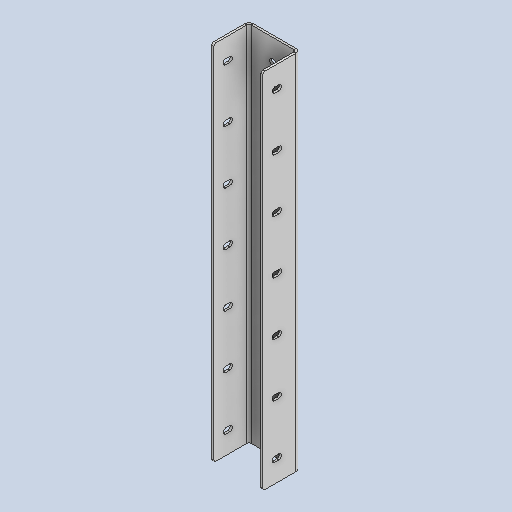
# Autodesk Inventor part: NDM 4.0.5  mother bottom
Saved by Autodesk Inventor 2025 (Build 290162010, 162A)
## iProperties
Created: 2023-07-04
Part Number: NDM 4.0.5  mother bottom
Material: Stainless Steel
Document SubType Name: Sheet Metal
Designer: user
Density: 8 g/cm^3
Sheet Metal Rule: Default_mm
Appearance: Default
Flat Pattern Width: 11.1048 cm
Flat Pattern Length: 34 cm
Flat Pattern Area: 377.562 cm^2
Sheet Metal Width: 111.048 mm
Sheet Metal Length: 340.000 mm
Sheet Metal Area: 37756.248 mm^2
Description: 2mm
Stock Number: NDM 4.0.5 мама низ
Mass: 594.459 g
Surface Area: 770.179 cm^2
Volume: 74.3073 cm^3
Author: user
Revision Number: 8
Autodesk Inventor part; units mm, degrees
ref_plane "YZ Plane" through (0, 0, 0) normal (1, 0, 0) x (0, 1, 0)
ref_plane "XZ Plane" through (0, 0, 0) normal (0, 1, 0) x (-1, 0, 0)
ref_plane "XY Plane" through (0, 0, 0) normal (0, 0, 1) x (1, 0, 0)
sketch "Sketch1" plane through (0, 0, 0) normal (0, 0, 1) x (1, 0, 0)
  line L0 (-22, 340) -> (22, 340)
  line L1 (22, 340) -> (22, 0)
  line L2 (22, 0) -> (-22, 0)
  line L3 (-22, 0) -> (-22, 340)
  line L4 (-22, 340) -> (22, 0) construction
  line L5 (22, 340) -> (-22, 0) construction
  point P0 (0, 0)
  point P1 (0, 170)
  point P2 (0, 0)
  dimension "d0" = 44
  dimension "d1" = 340
  constraints: 12 end point, 3 midpoint, 2 parallel, 1 coincident, 1 horizontal, 1 perpendicular
  measures "d0" distance of L1.end L2.end
  measures "d1" distance of L2.end L0.start
extrude "Plate1" add sketch "Sketch1" along normal blind 2
sketch "Sketch2" plane through (-22, 0, 2) normal (-1, 0, 0) x (0, -1, 0)
  line L0 (-340, 0) -> (0, 0)
  line L1 (0, 0) -> (0, 33)
  line L2 (0, 33) -> (-340, 33)
  line L3 (-340, 33) -> (-340, 0)
  constraints: 6 end point, 1 horizontal, 1 perpendicular, 1 vertical
edge flange "Flange1" height 35 angle 90 thickness 2 bend radius 2 thickness toward (-1, 0, 0) relief tear relief width 2 relief depth 1 corner gap 2 corner form 0 edges at (-22, 170, 2) (22, 170, 2) wall of the first edge with corners at (-22, 340, 2) (-22, 0, 2) (-22, 0, 35) (-22, 340, 35)
bend "Bend1"
corner "Corner1"
sketch "Sketch3" plane through (0, 0, 0) normal (1, 0, 0) x (0, 1, 0)
  line L0 (0, 4) -> (340, 4) projected
  line L1 (340, 35) -> (340, 4) projected
  line L2 (0, 35) -> (340, 35) projected
  line L3 (0, 4) -> (0, 35) projected
  circle A0 centre (20, 22) radius 2.5
  line L4 (20, 20) -> (20, 24) construction
  line L5 (22.5, 20) -> (22.5, 24)
  line L6 (17.5, 24) -> (17.5, 20)
  arc A1 (17.5, 20) -> (22.5, 20) centre (20, 20) ccw
  arc A2 (22.5, 24) -> (17.5, 24) centre (20, 24) ccw
  point P0 (0, 0)
  point P1 (17.5, 22)
  point P2 (22.5, 22)
  dimension "d13" = 5
  dimension "d14" = 13
  dimension "d15" = 20
  dimension "d28" = 4
  dimension "d29" = 2.5
  constraints: 8 end point, 4 point on circle, 4 tangent, 3 centre point, 1 coincident, 1 midpoint, 1 parallel, 1 vertical
  measures "d13" diameter of A0
  measures "d14" distance from line of A0.centre L2
  measures "d15" distance from line of L3 A0.centre
  measures "d28" distance of L4.start L4.end
  measures "d29" radius of A2
extrude "Extrusion1" cut sketch "Sketch3" along normal through all both and the other way through all contours A0 | L5 A1 L6 A0 | A0 L6 A2 L5
sketch "Sketch4" plane through (0, 0, 0) normal (0, 0, -1) x (-1, 0, 0)
  circle A0 centre (0, 20) radius 2.5
  line L0 (-20, 0) -> (20, 0) projected
  line L1 (-0.5, 20) -> (0.5, 20) construction
  line L2 (-0.5, 17.5) -> (0.5, 17.5)
  line L3 (0.5, 22.5) -> (-0.5, 22.5)
  arc A1 (-0.5, 22.5) -> (-0.5, 17.5) centre (-0.5, 20) ccw
  arc A2 (0.5, 17.5) -> (0.5, 22.5) centre (0.5, 20) ccw
  point P0 (0, 0)
  point P1 (0, 0)
  point P2 (0, 22.5)
  point P3 (0, 17.5)
  dimension "d21" = 5
  dimension "d22" = 20
  dimension "d30" = 1
  dimension "d31" = 5
  constraints: 8 end point, 4 point on circle, 4 tangent, 3 centre point, 2 midpoint, 1 coincident, 1 horizontal, 1 parallel, 1 vertical alignment
  measures "d21" diameter of A0
  measures "d22" distance from line of A0.centre L0
  measures "d30" distance of L1.start L1.end
  measures "d31" diameter of A2
extrude "Extrusion2" cut sketch "Sketch4" against normal through all
pattern_linear "Rectangular Pattern2" count 7 spacing 50 along (0, 1, 0) of "Extrusion2", "Extrusion1"
fillet "Fillet1" radius 2 4 edges at (-23, 0, 35) (23, 0, 35) (-23, 340, 35) (23, 340, 35)
equation "\"d22\" = d15"
equation "\"d2\" = Thickness"
equation "\"d3\" = BendReliefWidth"
equation "\"d4\" = BendReliefDepth"
equation "\"d5\" = MinimumRemnant"
equation "\"d6\" = TransitionRadius"
equation "\"d9\" = BendRadius"
equation "\"d10\" = CornerReliefSize"
equation "\"d11\" = GapSize"
equation "\"d12\" = JacobiRadiusSize"
equation "\"BendRadius\" = Thickness"
equation "\"BendReliefWidth\" = Thickness"
equation "\"BendReliefDepth\" = 0.5 * Thickness"
equation "\"CornerReliefSize\" = 4 * Thickness"
equation "\"MinimumRemnant\" = 2 * Thickness"
equation "\"TransitionRadius\" = BendRadius"
equation "\"JacobiRadiusSize\" = BendRadius"
equation "\"GapSize\" = Thickness"
equation "\"Thickness\" = 2"
body "Solid1"
